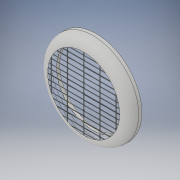
# Autodesk Inventor part: speakerGrill
Saved by Autodesk Inventor 2017 (Build 210142000, 142)
## iProperties
Created: 2018-08-03
Part Number: speakerGrill
Material: Generic
Document SubType Name: Modeling
Designer: Jake
Density: 1 g/cm^3
Appearance: Default
Author: Jake
Autodesk Inventor part; units mm, degrees
ref_plane "YZ Plane" through (0, 0, 0) normal (1, 0, 0) x (0, 1, 0)
ref_plane "XZ Plane" through (0, 0, 0) normal (0, 1, 0) x (-1, 0, 0)
ref_plane "XY Plane" through (0, 0, 0) normal (0, 0, 1) x (1, 0, 0)
sketch "Sketch1" plane through (0, 0, 0) normal (0, 0, 1) x (1, 0, 0)
  circle A0 centre (0, 0) radius 91.2813
  dimension "d0" = 182.5625
  constraints: 1 centre point, 1 coincident
  measures "d0" diameter of A0
extrude "Extrusion1" add sketch "Sketch1" along normal blind 25.4
fillet "Fillet1" radius 19.05 1 edges at (-91.2813, 0, 25.4)
shell "Shell1" thickness 17.78 removed faces 1 at (21.5393, 24.1816, 0)
body "Solid1"
